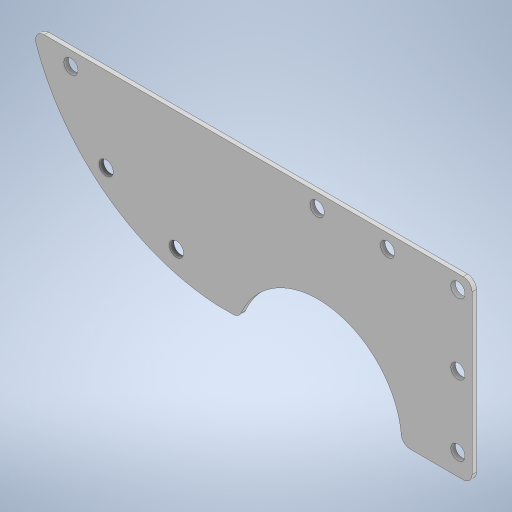
# Autodesk Inventor part: Horizontal climb
Saved by Autodesk Inventor 2023 (Build 270158000, 158)
## iProperties
Created: 2023-12-10
Part Number: Horizontal climb
Material: Generic
Document SubType Name: Modeling
Designer: diego
Density: 1 g/cm^3
Appearance: Default
Author: diego
Autodesk Inventor part; units mm, degrees
ref_plane "YZ Plane" through (0, 0, 0) normal (1, 0, 0) x (0, 1, 0)
ref_plane "XZ Plane" through (0, 0, 0) normal (0, 1, 0) x (-1, 0, 0)
ref_plane "XY Plane" through (0, 0, 0) normal (0, 0, 1) x (1, 0, 0)
sketch "Sketch1" plane through (0, 0, 0) normal (0, 0, 1) x (1, 0, 0)
  circle A0 centre (0, 0) radius 30.226
  line L0 (30.226, 0) -> (55.626, 0)
  line L1 (55.626, 0) -> (55.626, 63.5)
  line L2 (55.626, 63.5) -> (-103.124, 63.5)
  line L3 (-28.4673, 10.16) -> (-103.124, 10.16)
  line L4 (-103.124, 10.16) -> (-103.124, 63.5)
  arc A1 (-103.124, 63.5) -> (-28.4673, 10.16) centre (-32.2937, 83.7205) ccw
  point P0 (-36.1202, 10.16)
  dimension "d0" = 60.452
  dimension "d1" = 25.4
  dimension "d2" = 63.5
  dimension "d3" = 158.75
  dimension "d4" = 53.34
  dimension "d7" = 73.66
  constraints: 10 end point, 4 point on circle, 3 perpendicular, 2 centre point, 2 coincident, 1 horizontal, 1 parallel
  measures "d0" diameter of A0
  measures "d1" distance of L0.start L0.end
  measures "d2" distance of L0.end L1.end
  measures "d3" distance of L1.end L2.end
  measures "d4" distance of L3.end L2.end
  measures "d7" radius of A1
extrude "Extrusion1" add sketch "Sketch1" along normal blind 1.5875 contours A0 L3 A1 L2 L1 L0
sketch "Sketch2" plane through (0, 0, 1.5875) normal (0, 0, 1) x (1, 0, 0)
  line L0 (50.5354, 58.4509) -> (55.6154, 58.4509)
  line L1 (50.5354, 58.4509) -> (50.5354, 63.5309)
  circle A0 centre (50.5354, 58.4509) radius 2.54
  line L2 (50.5354, 58.4509) -> (50.5354, 33.0509)
  circle A1 centre (50.5354, 33.0509) radius 2.54
  line L3 (50.5354, 33.0509) -> (50.5354, 7.6509)
  circle A2 centre (50.5354, 7.6509) radius 2.54
  line L4 (50.5354, 58.4509) -> (25.1354, 58.4509)
  circle A3 centre (25.1354, 58.4509) radius 2.54
  line L5 (25.1354, 58.4509) -> (-0.2646, 58.4509)
  circle A4 centre (-0.2646, 58.4509) radius 2.54
  line L6 (-0.2646, 58.4509) -> (-89.1646, 58.4509)
  circle A5 centre (-89.1646, 58.4509) radius 2.54
  line L7 (50.5354, 33.0509) -> (-76.4646, 33.0509)
  circle A6 centre (-76.4646, 33.0509) radius 2.54
  line L8 (50.5354, 20.3509) -> (-51.0646, 20.3509)
  circle A7 centre (-51.0646, 20.3509) radius 2.54
  point P0 (0, 0)
  dimension "d16" = 5.08
  dimension "d17" = 25.4
  dimension "d18" = 5.08
  dimension "d19" = 25.4
  dimension "d20" = 5.08
  dimension "d21" = 25.4
  dimension "d22" = 5.08
  dimension "d23" = 25.4
  dimension "d24" = 5.08
  dimension "d25" = 88.9
  dimension "d26" = 5.08
  dimension "d29" = 127
  dimension "d30" = 5.08
  dimension "d31" = 101.6
  dimension "d32" = 5.08
  constraints: 18 end point, 8 centre point, 8 coincident, 5 horizontal, 3 vertical, 1 midpoint
  measures "d16" diameter of A0
  measures "d17" distance of L2.start L2.end
  measures "d18" diameter of A1
  measures "d19" distance of L3.start L3.end
  measures "d20" diameter of A2
  measures "d21" distance of L2.start L4.end
  measures "d22" diameter of A3
  measures "d23" distance of L5.start L5.end
  measures "d24" diameter of A4
  measures "d25" distance of L6.start L6.end
  measures "d26" diameter of A5
  measures "d29" distance of L3.start L7.end
  measures "d30" diameter of A6
  measures "d31" distance of L8.start L8.end
  measures "d32" diameter of A7
extrude "Extrusion2" cut sketch "Sketch2" against normal blind 25.4
fillet "Fillet1" radius 3.175 4 edges at (-103.124, 63.5, 0.7937) (55.626, 0, 0.7937) (30.226, 0, 0.7937) (55.626, 63.5, 0.7937)
fillet "Fillet2" radius 3.175 1 edges at (-28.4673, 10.16, 0.7937)
body "Solid1"
